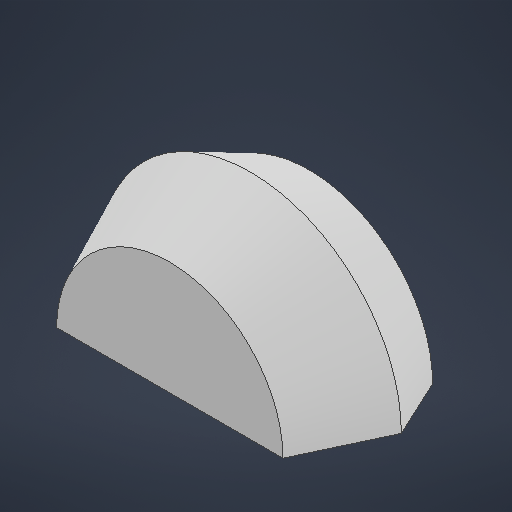
# Autodesk Inventor part: CUERPO_ABEJA
Saved by Autodesk Inventor 2026.2 (Build 302298000, 298)
## iProperties
Created: 2026-05-21
Part Number: CUERPO_ABEJA
Material: Generic
Document SubType Name: Modeling
Designer: juand
Density: 1 g/cm^3
Appearance: Default
Author: juand
Autodesk Inventor part; units mm, degrees
ref_plane "YZ Plane" through (0, 0, 0) normal (1, 0, 0) x (0, 1, 0)
ref_plane "XZ Plane" through (0, 0, 0) normal (0, 1, 0) x (-1, 0, 0)
ref_plane "XY Plane" through (0, 0, 0) normal (0, 0, 1) x (1, 0, 0)
sketch "Sketch1" plane through (0, 0, 0) normal (1, 0, 0) x (0, 1, 0)
  line L0 (0, 0) -> (57.3215, 15.3592)
  line L1 (57.3215, 15.3592) -> (70, 42.5485)
  line L2 (70, 42.5485) -> (52.5361, 80)
  line L3 (52.5361, 80) -> (0, 80)
  line L4 (0, 80) -> (0, 0)
  line L5 (51.899, 79) -> (68.8966, 42.5485)
  line L6 (68.8966, 42.5485) -> (56.6122, 16.2045)
  line L7 (56.6122, 16.2045) -> (1, 1.3032)
  line L8 (1, 1.3032) -> (1, 79)
  line L9 (1, 79) -> (51.899, 79)
  dimension "d0" = 90
  dimension "d1" = 75
  dimension "d2" = 130
  dimension "d3" = 130
  dimension "d4" = 80
  dimension "d5" = 70
  dimension "d6" = 30
  dimension "d7" = 1
  constraints: 20 end point, 1 vertical, 4 other
  measures "d0" angle of L4 L3
  measures "d1" angle of L0 L4
  measures "d2" angle of L0 L1
  measures "d3" angle of L2 L1
  measures "d4" distance of L3.end L0.start
  measures "d5" horizontal distance of L0.start L1.end
  measures "d6" distance of L0.end L1.end
  measures "d7" distance between parallel lines of L2 L5
revolve "Revolution1" add sketch "Sketch1" angle 180 mid plane about axis through (0, 0, 80) along (0, 0, -1)
body "Solid1"
